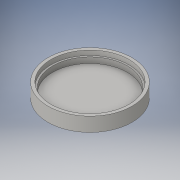
# Autodesk Inventor part: Soft Coating Gripper mold_6mil
Saved by Autodesk Inventor 2016 (Build 200138000, 138)
## iProperties
Created: 2017-10-13
Part Number: Soft Coating Gripper mold_6mil
Material: Generic
Document SubType Name: Modeling
Designer: ls769
Density: 1 g/cm^3
Appearance: Default
Author: ls769
Autodesk Inventor part; units mm, degrees
ref_plane "YZ Plane" through (0, 0, 0) normal (1, 0, 0) x (0, 1, 0)
ref_plane "XZ Plane" through (0, 0, 0) normal (0, 1, 0) x (-1, 0, 0)
ref_plane "XY Plane" through (0, 0, 0) normal (0, 0, 1) x (1, 0, 0)
sketch "Sketch4" plane through (0, 0, 0) normal (0, 1, 0) x (-1, 0, 0)
  circle A0 centre (0, 0) radius 39.75
  circle A1 centre (0, 0) radius 41.6215
  circle A2 centre (0, 0) radius 41.6213
  dimension "d17" = 79.5
  dimension "d18" = 83.243
  constraints: 3 centre point, 1 coincident
  measures "d17" diameter of A0
  measures "d18" diameter of A1
sketch "Sketch6" plane through (0, 0, 0) normal (0, 1, 0) x (-1, 0, 0)
  circle A0 centre (0, 0) radius 39.7618
  constraints: 1 centre point, 1 coincident
extrude "Extrusion1" add sketch "Sketch6" along normal blind 3
extrude "Extrusion2" add sketch "Sketch4" along normal blind 9
sketch "Sketch7" plane through (0, 0, 0) normal (0, -1, 0) x (1, 0, 0)
  circle A0 centre (0, 0) radius 44.86
  circle A1 centre (0, 0) radius 41.6213
  constraints: 2 centre point, 2 coincident
extrude "Extrusion3" add sketch "Sketch7" against normal blind 14
sketch "Sketch8" plane through (0, 0, 0) normal (0, -1, 0) x (1, 0, 0)
  circle A0 centre (0, 0) radius 44.86
  constraints: 1 centre point, 1 coincident
extrude "Extrusion4" add sketch "Sketch8" along normal blind 1
body "Solid1"
